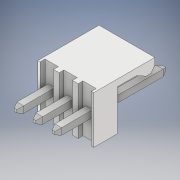
# Autodesk Inventor part: MOLEX_22-23-2031
Saved by Autodesk Inventor 2018 (Build 220112000, 112)
## iProperties
Created: 2018-01-14
Part Number: MOLEX_22-23-2031
Material: Generic
Document SubType Name: Modeling
Designer: jaden
Density: 1 g/cm^3
Appearance: Default
Author: jaden
Autodesk Inventor part; units mm, degrees
ref_plane "YZ Plane" through (0, 0, 0) normal (1, 0, 0) x (0, 1, 0)
ref_plane "XZ Plane" through (0, 0, 0) normal (0, 1, 0) x (-1, 0, 0)
ref_plane "XY Plane" through (0, 0, 0) normal (0, 0, 1) x (1, 0, 0)
sketch "Sketch1" plane through (0, 0, 0) normal (0, 0, 1) x (1, 0, 0)
  line L0 (-3.7338, -3.175) -> (3.7338, -3.175)
  line L1 (3.7338, -3.175) -> (3.7338, 3.175)
  line L2 (3.7338, 3.175) -> (-3.7338, 3.175)
  line L3 (-3.7338, 3.175) -> (-3.7338, -3.175)
  line L4 (-2.54, 3.175) -> (-2.54, -3.175) construction
  line L5 (-3.7338, 0.0762) -> (3.7338, 0.0762) construction
  line L6 (0, 3.175) -> (0, -3.175) construction
  line L7 (2.54, 3.175) -> (2.54, -3.175) construction
  line L8 (-2.9845, -0.3683) -> (-2.0955, -0.3683)
  line L9 (-2.0955, -0.3683) -> (-2.0955, 0.5207)
  line L10 (-2.0955, 0.5207) -> (-2.9845, 0.5207)
  line L11 (-2.9845, 0.5207) -> (-2.9845, -0.3683)
  line L12 (-0.4445, -0.3683) -> (0.4445, -0.3683)
  line L13 (0.4445, -0.3683) -> (0.4445, 0.5207)
  line L14 (0.4445, 0.5207) -> (-0.4445, 0.5207)
  line L15 (-0.4445, 0.5207) -> (-0.4445, -0.3683)
  line L16 (2.0955, -0.3683) -> (2.9845, -0.3683)
  line L17 (2.9845, -0.3683) -> (2.9845, 0.5207)
  line L18 (2.9845, 0.5207) -> (2.0955, 0.5207)
  line L19 (2.0955, 0.5207) -> (2.0955, -0.3683)
  point P0 (-2.54, 0.0762)
  point P1 (0, 0.0762)
  point P2 (2.54, 0.0762)
  dimension "d0" = 6.35
  dimension "d1" = 7.4676
  dimension "d2" = 1.1938
  dimension "d3" = 3.0988
  dimension "d4" = 1.1938
  dimension "d5" = 2.54
  dimension "d6" = 0.889
  dimension "d7" = 0.889
  dimension "d8" = 0.889
  dimension "d9" = 0.889
  dimension "d10" = 0.889
  dimension "d11" = 0.889
  constraints: 40 end point, 11 point on line, 8 parallel, 8 perpendicular, 4 horizontal, 3 midpoint
  measures "d0" distance between parallel lines of L0 L2
  measures "d1" distance between parallel lines of L3 L1
  measures "d2" distance between parallel lines of L4 L3
  measures "d3" distance between parallel lines of L2 L5
  measures "d4" distance between parallel lines of L1 L7
  measures "d5" distance between parallel lines of L4 L6
  measures "d6" distance of L10.end L9.end
  measures "d7" distance of L9.end L8.end
  measures "d8" distance of L14.end L13.end
  measures "d9" distance of L13.end L12.end
  measures "d10" distance of L18.end L17.end
  measures "d11" distance of L17.end L16.end
extrude "Extrusion1" add sketch "Sketch1" along normal blind 3.175
sketch "Sketch16" plane through (-3.7338, -3.175, 0) normal (0, -1, 0) x (1, 0, 0)
  line L0 (7.4676, 3.175) -> (0, 3.175)
  line L1 (7.1628, 3.175) -> (5.3848, 3.175)
  line L2 (5.3848, 3.175) -> (5.3848, 2.5324)
  line L3 (5.3848, 2.5324) -> (7.1628, 2.5324)
  line L4 (7.1628, 2.5324) -> (7.1628, 3.175)
  line L5 (2.8448, 2.5324) -> (4.6228, 2.5324)
  line L6 (4.6228, 2.5324) -> (4.6228, 3.175)
  line L7 (4.6228, 3.175) -> (2.8448, 3.175)
  line L8 (2.8448, 3.175) -> (2.8448, 2.5324)
  line L9 (0.3048, 2.5324) -> (2.0828, 2.5324)
  line L10 (2.0828, 2.5324) -> (2.0828, 3.175)
  line L11 (2.0828, 3.175) -> (0.3048, 3.175)
  line L12 (0.3048, 3.175) -> (0.3048, 2.5324)
  line L13 (7.4676, 0) -> (7.4676, 3.175)
  line L14 (0, 0) -> (0, 3.175)
  line L15 (7.1628, 2.5324) -> (5.3848, 2.5324)
  line L16 (5.3848, 2.5324) -> (5.3848, 3.175)
  line L17 (5.3848, 3.175) -> (7.1628, 3.175)
  line L18 (7.1628, 3.175) -> (7.1628, 2.5324)
  point P0 (3.7338, 0)
  point P1 (3.7338, 0)
  dimension "d103" = 1.778
  dimension "d104" = 0.6426
  dimension "d105" = 2.54
  dimension "d106" = 0.3048
  dimension "d107" = 0.3048
  constraints: 38 end point, 4 parallel, 3 horizontal, 2 perpendicular, 1 point on line, 16 other
  measures "d103" distance of L3.end L2.end
  measures "d104" distance of L2.end L1.end
  measures "d105" distance of L2.end L5.start
  measures "d106" distance between parallel lines of L13 L4
  measures "d107" distance between parallel lines of L14 L12
extrude "Extrusion8" cut sketch "Sketch16" against normal through all
sketch "Sketch2" plane through (0, 0, 0) normal (0, 0, -1) x (-1, 0, 0)
  line L0 (-3.7338, -3.175) -> (3.7338, -3.175)
  line L1 (3.7338, -3.175) -> (3.7338, 3.175)
  line L2 (3.7338, 3.175) -> (-3.7338, 3.175)
  line L3 (-3.7338, 3.175) -> (-3.7338, -3.175)
  line L4 (-2.54, 3.175) -> (-2.54, -3.175) construction
  line L5 (-3.7338, 0.0762) -> (3.7338, 0.0762) construction
  line L6 (0, 3.175) -> (0, -3.175) construction
  line L7 (2.54, 3.175) -> (2.54, -3.175) construction
  line L8 (-2.9845, -0.3683) -> (-2.0955, -0.3683)
  line L9 (-2.0955, -0.3683) -> (-2.0955, 0.5207)
  line L10 (-2.0955, 0.5207) -> (-2.9845, 0.5207)
  line L11 (-2.9845, 0.5207) -> (-2.9845, -0.3683)
  line L12 (-0.4445, -0.3683) -> (0.4445, -0.3683)
  line L13 (0.4445, -0.3683) -> (0.4445, 0.5207)
  line L14 (0.4445, 0.5207) -> (-0.4445, 0.5207)
  line L15 (-0.4445, 0.5207) -> (-0.4445, -0.3683)
  line L16 (2.0955, -0.3683) -> (2.9845, -0.3683)
  line L17 (2.9845, -0.3683) -> (2.9845, 0.5207)
  line L18 (2.9845, 0.5207) -> (2.0955, 0.5207)
  line L19 (2.0955, 0.5207) -> (2.0955, -0.3683)
  point P0 (0, 0)
  point P1 (-2.54, 0.0762)
  point P2 (0, 0.0762)
  point P3 (2.54, 0.0762)
  dimension "d14" = 6.35
  dimension "d15" = 7.4676
  dimension "d16" = 1.1938
  dimension "d17" = 3.0988
  dimension "d18" = 1.1938
  dimension "d19" = 2.54
  dimension "d20" = 0.889
  dimension "d21" = 0.889
  dimension "d22" = 0.889
  dimension "d23" = 0.889
  dimension "d24" = 0.889
  dimension "d25" = 0.889
  constraints: 40 end point, 11 point on line, 8 parallel, 8 perpendicular, 4 horizontal, 3 midpoint
  measures "d14" distance between parallel lines of L0 L2
  measures "d15" distance between parallel lines of L3 L1
  measures "d16" distance between parallel lines of L4 L3
  measures "d17" distance between parallel lines of L2 L5
  measures "d18" distance between parallel lines of L1 L7
  measures "d19" distance between parallel lines of L4 L6
  measures "d20" distance of L10.end L9.end
  measures "d21" distance of L9.end L8.end
  measures "d22" distance of L14.end L13.end
  measures "d23" distance of L13.end L12.end
  measures "d24" distance of L18.end L17.end
  measures "d25" distance of L17.end L16.end
extrude "Extrusion2" add sketch "Sketch2" along normal blind 6.858 and the other way blind 6.731 contours L11 L10 L9 L8 | L15 L14 L13 L12 | L19 L18 L17 L16
sketch "Sketch3" plane through (0, 0, -6.858) normal (0, 0, -1) x (-1, 0, 0)
  line L0 (-2.54, 0.5207) -> (-2.54, -0.3683) construction
  line L1 (-2.0955, 0.0762) -> (-2.9845, 0.0762) construction
  line L2 (-2.7337, -0.1143) -> (-2.3463, -0.1143)
  line L3 (-2.3463, -0.1143) -> (-2.3463, 0.2667)
  line L4 (-2.3463, 0.2667) -> (-2.7337, 0.2667)
  line L5 (-2.7337, 0.2667) -> (-2.7337, -0.1143)
  line L6 (-2.7337, -0.1143) -> (-2.3463, 0.2667) construction
  line L7 (-2.3463, -0.1143) -> (-2.7337, 0.2667) construction
  point P0 (0, 0)
  point P1 (-2.54, 0.0762)
  dimension "d30" = 0.381
  constraints: 16 end point, 3 midpoint, 2 parallel, 1 horizontal, 1 perpendicular
  measures "d30" distance of L3.end L2.end
extrude "Extrusion3" add sketch "Sketch3" along normal blind 0.635
loft "Loft1" add section 1 edges at (2.54, -0.3683, -6.858) (2.0955, 0.0762, -6.858) (2.54, 0.5207, -6.858) (2.9845, 0.0762, -6.858) section 2 edges at (2.54, -0.1143, -7.493) (2.3463, 0.0762, -7.493) (2.54, 0.2667, -7.493) (2.7337, 0.0762, -7.493)
sketch "Sketch12" plane through (3.7338, -3.175, 0) normal (1, 0, 0) x (0, 0, -1)
  line L0 (0, 0) -> (0, 6.35) construction
  line L1 (0, 5.0165) -> (-3.1732, 5.0165) construction
  line L2 (0, 6.35) -> (-3.175, 6.35) construction
  line L3 (0, 6.35) -> (0, 0) projected
  line L4 (0, 6.35) -> (5.0038, 6.35)
  line L5 (5.0038, 6.35) -> (5.0038, 5.461)
  line L6 (2.5019, 5.461) -> (0, 5.461)
  line L7 (0, 5.461) -> (0, 6.35)
  line L8 (5.0038, 5.461) -> (4.4958, 4.7625)
  line L9 (4.4958, 4.7625) -> (3.8608, 4.7625)
  line L10 (0, 3.6957) -> (6.858, 3.6957) projected
  line L11 (3.8608, 4.7625) -> (2.5019, 5.461)
  point P0 (0, 3.175)
  dimension "d57" = 1.3335
  dimension "d58" = 5.0038
  dimension "d59" = 0.889
  dimension "d60" = 1.0668
  dimension "d61" = 2.5019
  dimension "d62" = 0.508
  dimension "d63" = 0.635
  constraints: 16 end point, 3 horizontal, 2 parallel, 1 perpendicular, 1 point on line
  measures "d57" distance between parallel lines of L2 L1
  measures "d58" distance of L5.end L6.end
  measures "d59" distance of L4.end L5.end
  measures "d60" distance between parallel lines of L10 L9
  measures "d61" distance from line of L5 L6.start
  measures "d62" horizontal distance of L4.end L8.end
  measures "d63" distance of L8.end L9.end
extrude "Extrusion6" add sketch "Sketch12" against normal blind 7.4676
sketch "Sketch6" plane through (0, 0, 6.731) normal (0, 0, 1) x (1, 0, 0)
  line L0 (2.54, -0.3683) -> (2.54, 0.5207) construction
  line L1 (2.7305, 0.2667) -> (2.3495, 0.2667)
  line L2 (2.3495, 0.2667) -> (2.3495, -0.1143)
  line L3 (2.3495, -0.1143) -> (2.7305, -0.1143)
  line L4 (2.7305, -0.1143) -> (2.7305, 0.2667)
  line L5 (2.7305, 0.2667) -> (2.3495, -0.1143) construction
  line L6 (2.3495, 0.2667) -> (2.7305, -0.1143) construction
  point P0 (0, 0)
  point P1 (2.54, 0.0762)
  dimension "d37" = 0.381
  dimension "d38" = 0.381
  constraints: 14 end point, 2 midpoint, 2 parallel, 1 horizontal, 1 perpendicular
  measures "d37" distance of L3.end L2.end
  measures "d38" distance of L2.end L1.end
extrude "Extrusion4" add sketch "Sketch6" along normal blind 0.635
loft "Loft2" add section 1 edges at (2.54, -0.3683, 6.731) (2.9845, 0.0762, 6.731) (2.54, 0.5207, 6.731) (2.0955, 0.0762, 6.731) section 2 edges at (2.54, 0.2667, 7.366) (2.3495, 0.0762, 7.366) (2.54, -0.1143, 7.366) (2.7305, 0.0762, 7.366)
pattern_linear "Rectangular Pattern1" count 3 spacing 2.54 along (-1, 0, 0) of "Loft1"
pattern_linear "Rectangular Pattern2" count 3 spacing 2.54 along (-1, 0, 0) of "Loft2"
body "Solid1"
